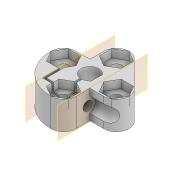
# Autodesk Inventor part: sonic hub 1_4 D 3mm
Saved by Autodesk Inventor 2020 (Build 240168000, 168)
## iProperties
Created: 2019-12-14
Part Number: sonic hub 1_4 D 3mm
Material: Generic
Document SubType Name: Modeling
Designer: ball
Density: 1 g/cm^3
Appearance: Default
Author: ball
Autodesk Inventor part; units mm, degrees
ref_plane "YZ Plane" through (0, 0, 0) normal (1, 0, 0) x (0, 1, 0)
ref_plane "XZ Plane" through (0, 0, 0) normal (0, 1, 0) x (-1, 0, 0)
ref_plane "XY Plane" through (0, 0, 0) normal (0, 0, 1) x (1, 0, 0)
sketch "Sketch1" plane through (0, 0, 0) normal (0, 1, 0) x (-1, 0, 0)
  circle A0 centre (9.779, 0) radius 1.9304
  line L0 (0, 9.779) -> (0, 0) construction
  line L1 (9.779, 0) -> (0, 0) construction
  arc A1 (-2.5908, -2.0472) -> (-2.5908, 2.0472) centre (0, 0) ccw
  line L2 (-2.5908, 2.0472) -> (-2.5908, -2.0472)
  circle A2 centre (0, 9.779) radius 1.9304
  circle A3 centre (-9.779, 0) radius 1.9304
  circle A4 centre (0, -9.779) radius 1.9304
  line L3 (4.7625, 7.21) -> (-2.8575, 7.21) construction
  line L4 (-2.8575, 7.21) -> (-2.8575, 3.81) construction
  line L5 (-2.8575, 3.81) -> (4.7625, 3.81) construction
  line L6 (4.7625, 3.81) -> (4.7625, 7.21) construction
  line L7 (4.7625, 8.2835) -> (7.5625, 8.2835) construction
  line L8 (7.5625, 8.2835) -> (7.5625, 2.3835) construction
  line L9 (7.5625, 2.3835) -> (4.7625, 2.3835) construction
  line L10 (4.7625, 2.3835) -> (4.7625, 8.2835) construction
  circle A5 centre (0, -9.779) radius 4.6609 construction
  circle A6 centre (0, 9.779) radius 4.6609 construction
  circle A7 centre (9.779, 0) radius 4.6609 construction
  circle A8 centre (-9.779, 0) radius 4.6609 construction
  line L11 (-4.6609, 9.779) -> (-4.6609, -11.7096) construction
  line L12 (-9.779, 4.6609) -> (-4.6609, 4.6609)
  line L13 (-13.0748, -3.2958) -> (-3.2958, -13.0748)
  line L14 (4.6609, -9.779) -> (4.6609, 9.779) construction
  line L15 (9.779, -4.6609) -> (4.6609, -4.6609)
  line L16 (4.6609, -9.779) -> (4.6609, -4.6609)
  arc A9 (-9.779, 4.6609) -> (-13.0748, -3.2958) centre (-9.779, 0) ccw
  arc A10 (-3.2958, -13.0748) -> (4.6609, -9.779) centre (0, -9.779) ccw
  line L17 (-4.6609, 9.779) -> (-4.6609, 4.6609)
  arc A11 (14.4399, 0) -> (0, 14.4399) centre (0, 0) ccw
  arc A12 (0, 14.4399) -> (-4.6609, 9.779) centre (0, 9.779) ccw
  arc A13 (9.779, -4.6609) -> (14.4399, 0) centre (9.779, 0) ccw
  point P0 (-13.0748, -3.2958)
  dimension "d0" = 3.8608
  dimension "d2" = 0
  dimension "d3" = 9.779
  dimension "d12" = 6.604
  dimension "d13" = 2.5908
  dimension "d16" = 360
  dimension "d18" = 7.62
  dimension "d19" = 3.4
  dimension "d20" = 3.81
  dimension "d21" = 2.8
  dimension "d22" = 5.9
  dimension "d23" = 9.3218
  dimension "d24" = 9.3218
  dimension "d25" = 9.3218
  dimension "d26" = 9.3218
  constraints: 36 end point, 22 point on circle, 14 centre point, 10 coincident, 8 tangent, 4 parallel, 4 perpendicular, 3 point on line, 3 vertical, 2 collinear, 2 concentric, 2 horizontal, 9 other
  measures "d0" diameter of A0
  measures "d2" vertical distance of L0.end A0.centre
  measures "d3" distance of L0.end A0.centre
  measures "d12" diameter of A1
  measures "d13" distance from line of L2 L0.end
  measures "d18" distance of L5.end L4.end
  measures "d19" distance of L4.end L3.end
  measures "d20" distance from line of L0.end L5
  measures "d21" distance of L8.end L9.end
  measures "d22" distance of L7.end L8.end
  measures "d23" diameter of A5
  measures "d24" diameter of A6
  measures "d25" diameter of A7
  measures "d26" diameter of A8
extrude "Extrusion1" add sketch "Sketch1" along normal mid plane 10.4
sketch "Sketch2" plane through (0, 5.2, 0) normal (0, 1, 0) x (1, 0, 0)
  circle A0 centre (-9.779, 0) radius 1.9304 construction
  circle A1 centre (-9.779, 0) radius 4.6609 construction
  line L0 (-14.4399, 0) -> (-12.1095, 4.0365)
  line L1 (-12.1095, 4.0365) -> (-7.4486, 4.0365)
  line L2 (-7.4486, 4.0365) -> (-5.1181, 0)
  line L3 (-5.1181, 0) -> (-7.4485, -4.0365)
  line L4 (-7.4485, -4.0365) -> (-12.1094, -4.0365)
  line L5 (-12.1094, -4.0365) -> (-14.4399, 0)
  circle A2 centre (0, -9.779) radius 4.6609 construction
  line L6 (0, -14.4399) -> (-4.0365, -12.1095)
  line L7 (-4.0365, -12.1095) -> (-4.0365, -7.4486)
  line L8 (-4.0365, -7.4486) -> (0, -5.1181)
  line L9 (0, -5.1181) -> (4.0365, -7.4485)
  line L10 (4.0365, -7.4485) -> (4.0365, -12.1094)
  line L11 (4.0365, -12.1094) -> (0, -14.4399)
  circle A3 centre (9.779, 0) radius 4.6609 construction
  line L12 (14.4399, 0) -> (12.1095, -4.0365)
  line L13 (12.1095, -4.0365) -> (7.4486, -4.0365)
  line L14 (7.4486, -4.0365) -> (5.1181, 0)
  line L15 (5.1181, 0) -> (7.4485, 4.0365)
  line L16 (7.4485, 4.0365) -> (12.1094, 4.0365)
  line L17 (12.1094, 4.0365) -> (14.4399, 0)
  circle A4 centre (0, 9.779) radius 4.6609 construction
  line L18 (0, 14.4399) -> (4.0365, 12.1095)
  line L19 (4.0365, 12.1095) -> (4.0365, 7.4485)
  line L20 (4.0365, 7.4485) -> (0, 5.1181)
  line L21 (0, 5.1181) -> (-4.0365, 7.4485)
  line L22 (-4.0365, 7.4485) -> (-4.0365, 12.1094)
  line L23 (-4.0365, 12.1094) -> (0, 14.4399)
  point P0 (0, 0)
  dimension "d29" = 9.3218
  dimension "d32" = 360
  constraints: 48 end point, 8 coincident, 2 horizontal alignment, 2 vertical alignment, 86 other
extrude "Extrusion2" cut sketch "Sketch2" against normal blind 3.048
ref_plane "Work Plane1" through (4.6609, 0, 9.779) normal (1, 0, 0) x (0, 1, 0)
sketch "Sketch3" plane through (4.6609, 0, 9.779) normal (1, 0, 0) x (0, 1, 0)
  line L0 (2.152, -1.9304) -> (-5.2, -1.9304) construction
  line L1 (5.2, -6.477) -> (-5.2, -6.477) construction
  point P0 (0, -9.779)
  point P1 (0, -4.2037)
  dimension "d36" = 4.5466
  dimension "d37" = 2.2733
  measures "d36" distance between parallel lines of L1 L0
  measures "d37" distance from line of L0 point (0, -4.204)
hole "Hole1" at (4.6609, 0, 5.5753) direction (-1, 0, 0) diameter 3.4 depth 12
sketch "Sketch4" plane through (4.6609, 0, 9.779) normal (1, 0, 0) x (0, 1, 0)
  circle A0 centre (0, -4.2037) radius 1.7 projected
  circle A1 centre (0, -4.2037) radius 2.95
  point P0 (0, -9.779)
  dimension "d45" = 5.9
  constraints: 1 centre point, 1 coincident
  measures "d45" diameter of A1
extrude "Extrusion3" cut sketch "Sketch4" along normal blind 10.4 contours A0 | A1
sketch "Sketch6" plane through (0, -5.2, 0) normal (0, -1, 0) x (1, 0, 0)
  line L0 (-7.3391, 7.2753) -> (4.6609, 7.2753) construction
  line L1 (-7.3391, 3.8753) -> (4.6609, 3.8753) construction
  point P0 (0, 0)
ref_plane "Work Plane2" through (-7.3391, 0, 9.779) normal (1, 0, 0) x (0, 1, 0)
sketch "Sketch7" plane through (-7.3391, 0, 9.779) normal (1, 0, 0) x (0, 1, 0)
  circle A0 centre (0, -4.2037) radius 1.7 construction
  circle A1 centre (0, -4.2037) radius 3.45 construction
  line L0 (3.45, -4.2037) -> (1.725, -7.1915)
  line L1 (5.175, -7.1915) -> (-5.2, -7.1915)
  line L2 (-5.2, -1.2159) -> (1.725, -1.2159)
  line L3 (1.725, -1.2159) -> (3.45, -4.2037)
  line L4 (-5.2, 4.6609) -> (-5.2, -9.779) projected
  line L5 (-5.2, -1.2159) -> (-5.2, -7.1915)
  point P0 (0, -9.779)
  dimension "d49" = 6.9
  constraints: 10 end point, 4 point on line, 2 coincident, 1 horizontal alignment, 1 perpendicular, 8 other
extrude "Extrusion4" cut sketch "Sketch7" against normal blind 2
sketch "Sketch8" plane through (0, -5.2, 0) normal (0, -1, 0) x (1, 0, 0)
  line L0 (0.3175, 0) -> (0.3175, 9.779)
  line L1 (0.3175, 9.779) -> (-0.3175, 9.779)
  line L2 (-0.3175, 9.779) -> (-0.3175, 0)
  line L3 (-0.3175, -9.779) -> (0.3175, 9.779) construction
  line L4 (0.3175, -9.779) -> (-0.3175, 9.779) construction
  line L5 (-0.3175, 0) -> (0.3175, 0)
  line L6 (-7.3391, 20.2159) -> (-7.3391, -20.2159) construction
  line L7 (0.3175, 9.4615) -> (-7.3391, 9.4615)
  line L8 (-7.3391, 9.4615) -> (-7.3391, 10.0965)
  line L9 (-7.3391, 10.0965) -> (0.3175, 10.0965)
  line L10 (3.348, 9.6342) -> (-7.3391, 10.0965) construction
  line L11 (-7.3391, 9.4615) -> (3.348, 9.9238) construction
  line L12 (0.3175, 9.4615) -> (0.3175, 10.0965)
  line L13 (-7.3391, 10.0965) -> (-6.7041, 10.0965)
  line L14 (-6.7041, 10.0965) -> (-6.7041, 0)
  line L15 (-6.7041, 0) -> (-7.3391, 0)
  line L16 (-7.3391, 0) -> (-7.3391, 10.0965)
  point P0 (0, 0)
  point P1 (0, 9.779)
  point P2 (-6.7041, 9.4615)
  point P3 (-0.3175, 9.4615)
  dimension "d52" = 0.635
  dimension "d53" = 0.635
  dimension "d54" = 0.635
  constraints: 32 end point, 5 point on line, 4 parallel, 3 midpoint, 2 horizontal, 2 perpendicular, 1 vertical
  measures "d52" distance of L1.end L0.end
  measures "d53" distance of L7.end L8.end
  measures "d54" distance of L14.end L15.end
extrude "Extrusion5" cut sketch "Sketch8" against normal through all
equation "\"d23\" = d24"
equation "\"d25\" = d24"
equation "\"d26\" = d24"
equation "\"d37\" = 0.5 * d36"
body "Solid1"
